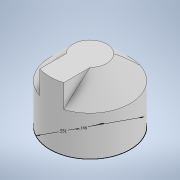
# Autodesk Inventor part: knob
Saved by Autodesk Inventor 2020 (Build 240168000, 168)
## iProperties
Created: 2022-01-22
Part Number: knob
Material: Generic
Document SubType Name: Modeling
Designer: gamma
Density: 1 g/cm^3
Appearance: Default
Author: gamma
Autodesk Inventor part; units mm, degrees
ref_plane "YZ Plane" through (0, 0, 0) normal (1, 0, 0) x (0, 1, 0)
ref_plane "XZ Plane" through (0, 0, 0) normal (0, 1, 0) x (-1, 0, 0)
ref_plane "XY Plane" through (0, 0, 0) normal (0, 0, 1) x (1, 0, 0)
sketch "Sketch1" plane through (0, 0, 0) normal (0, 1, 0) x (-1, 0, 0)
  circle A0 centre (0, 0) radius 1.85
  circle A1 centre (0, 0) radius 7
  line L0 (-2.101008, -6.677257) -> (-2.101008, 6.677257)
  line L1 (-2.101008, 6.677257) -> (2.101008, 6.677257)
  line L2 (2.101008, 6.677257) -> (2.101008, -6.677257)
  line L3 (2.101008, -6.677257) -> (-2.101008, -6.677257)
  line L4 (-2.101008, -6.677257) -> (2.101008, 6.677257) construction
  line L5 (-2.101008, 6.677257) -> (2.101008, -6.677257) construction
  line L6 (2.101008, 0) -> (-2.101008, 0)
  point P0 (-1.841091, -0.181341)
  point P1 (1.841091, 0.181341)
  point P2 (2.101008, -6.677257)
  point P3 (1.85, 6.751111)
  point P4 (-2.101008, -6.677257)
  point P5 (2.101008, -6.677257)
  point P6 (-2.101008, 6.677257)
  dimension "d1" = 14
  dimension "d0" = 3.7
  constraints: 14 end point, 4 midpoint, 2 coincident, 2 parallel, 1 centre point, 1 perpendicular, 1 vertical, 3 other
  measures "d0" diameter of A0
extrude "Extrusion1" add sketch "Sketch1" along normal blind 11 contours L2 A1 | L0 A1
chamfer "Chamfer1" distance 4.064 angle 45 2 edges at (-7, 11, 0) (7, 11, 0)
extrude "Extrusion2" add sketch "Sketch1" along normal blind 11 contours L6 L2 L3 L0 A0 | A0 L6 L0 L1 L2
extrude "Extrusion3" add sketch "Sketch1" along normal blind 11.000003 contours A1 L3
chamfer "Chamfer2" distance 4.064 angle 45 1 edges at (0, 11, -7)
extrude "Extrusion4" add sketch "Sketch1" along normal blind 11.000003 contours L6 A0 | A0 L6
extrude "Extrusion5" cut sketch "Sketch1" along normal blind 7.9 contours L6 A0 | A0 L6
extrude "Extrusion6" add sketch "Sketch1" along normal blind 11 contours L1 A1
body "Solid1"
